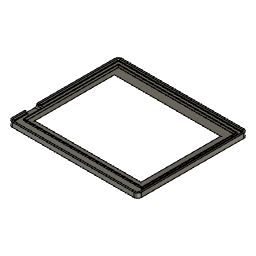
Soldered Inkplate 6Color v1.2.0. Case (Autodesk Fusion 360 archive; units mm, degrees)
design "Inkplate 6Color v1.2.0. Top"
Autodesk Fusion 360 part; units mm, degrees
sketch "Sketch1" plane through (0, 0, 0) normal (0, 0, 1) x (1, 0, 0)
  line L0 (70.2, 58.7) -> (-70.2, 58.7)
  line L1 (-70.2, 58.7) -> (-70.2, -60.7)
  line L2 (-70.2, -60.7) -> (70.2, -60.7)
  line L3 (70.2, -60.7) -> (70.2, 58.7)
  line L4 (0, 0) -> (0, -1) construction
  line L5 (58.2, 42.8) -> (-58.2, 42.8)
  line L6 (-58.2, 42.8) -> (-58.2, -44.8)
  line L7 (-58.2, -44.8) -> (58.2, -44.8)
  line L8 (58.2, -44.8) -> (58.2, 42.8)
  line L9 (58.2, 42.8) -> (-58.2, -44.8) construction
  line L10 (-58.2, 42.8) -> (58.2, -44.8) construction
  line L11 (-63.45, 47.4) -> (63.45, 47.4)
  line L12 (63.45, 47.4) -> (63.45, -52.1)
  line L13 (63.45, -52.1) -> (-63.45, -52.1)
  line L14 (-63.45, -52.1) -> (-63.45, 47.4)
  line L15 (57.6, 42.8) -> (57.6, -44.8)
  line L16 (58.2, 42.15) -> (-58.2, 42.15)
  line L17 (58.2, -44.5) -> (-58.2, -44.5)
  line L18 (-57.95, -44.8) -> (-57.95, 42.8)
  point P0 (0, -1)
  dimension "d1" = 140.4
  dimension "d55" = 1
  dimension "d56" = 116.4
  dimension "d57" = 87.6
  dimension "d58" = 15.9
  dimension "d59" = 15.9
  dimension "d60" = 119.4
  dimension "d61" = 4.6
  dimension "d62" = 5.25
  dimension "d63" = 5.25
  dimension "d64" = 99.5
  dimension "d67" = 0.6
  dimension "d68" = 0.65
  dimension "d69" = 0.25
  dimension "d70" = 0.3
  constraint horizontal L0
  constraint perpendicular L0 L1
  constraint parallel L0 L2
  constraint parallel L1 L3
  constraint coincident L4.start origin
  constraint vertical L4
  constraint horizontal L5
  constraint perpendicular L5 L6
  constraint parallel L5 L7
  constraint parallel L6 L8
  constraint coincident L9 P0
  constraint coincident L10 P0
  constraint coincident P0 L4.end
  constraint horizontal L11
  constraint vertical L12
  constraint horizontal L13
  constraint vertical L14
  constraint coincident L5 L15.start
  constraint coincident L7 L15.end
  constraint perpendicular L7 L15
  constraint coincident L8 L16.start
  constraint coincident L6 L16.end
  constraint perpendicular L6 L16
  constraint coincident L8 L17.start
  constraint coincident L6 L17.end
  constraint perpendicular L6 L17
  constraint coincident L7 L18.start
  constraint coincident L5 L18.end
  constraint perpendicular L5 L18
  measures "d1" distance of L1.end L2.end
  measures "d55" distance of L4.start P0
  measures "d56" distance of L6.end L7.end
  measures "d57" distance of L5.end L6.end
  measures "d58" distance of L0 L5
  measures "d59" distance of L2 L7
  measures "d60" distance of L0.end L1.end
  measures "d61" distance of L5 L11
  measures "d62" distance of L6 L14
  measures "d63" distance of L8 L12
  measures "d64" distance of L11.start L13.end
  measures "d67" distance of L8 L15
  measures "d68" distance of L5 L16
  measures "d69" distance of L6 L18
  measures "d70" distance of L7 L17
extrude "Extrude1" add sketch "Sketch1" along normal blind 5 contours L0 L1 L2 L3 | L5 L8 L15 L16 | L5 L15 L16 L18 | L8 L15 L16 L17 | L5 L6 L16 L18 | L7 L8 L15 L17 | L6 L16 L17 L18 | L7 L15 L17 L18 | L6 L7 L17 L18 | L11 L12 L13 L14
sketch "Sketch2" plane through (0, 0, 5) normal (0, 0, 1) x (-1, 0, 0)
  line L0 (70.2, 60.7) -> (-70.2, 60.7)
  line L1 (68.6, -57.1) -> (-68.6, -57.1)
  line L2 (-68.6, -57.1) -> (-68.6, 59.1)
  line L3 (-68.6, 59.1) -> (68.6, 59.1)
  line L4 (68.6, 59.1) -> (68.6, -57.1)
  line L5 (70.2, -58.7) -> (70.2, 60.7)
  line L6 (-70.2, -58.7) -> (70.2, -58.7)
  line L7 (-70.2, 60.7) -> (-70.2, -58.7)
  dimension "d71" = 1.6
  dimension "d72" = 1.6
  dimension "d73" = 1.6
  dimension "d74" = 1.6
  constraint horizontal L1
  constraint vertical L2
  constraint horizontal L3
  constraint vertical L4
  measures "d71" distance of L4 L5
  measures "d72" distance of L1 L6
  measures "d73" distance of L2 L7
  measures "d74" distance of L0 L3
extrude "Extrude2" cut sketch "Sketch2" against normal blind 3 contours L1 L2 L3 L4
chamfer "Chamfer1" distance 2 angle 45 4 edges at (-0.175, 42.15, 0) (57.6, -1.175, 0) (-0.175, -44.5, 0) (-57.95, -1.175, 0)
fillet "Fillet1" radius 4 4 edges at (70.2, -60.7, 2.5) (-70.2, -60.7, 2.5) (-70.2, 58.7, 2.5) (70.2, 58.7, 2.5)
sketch "Sketch3" plane through (0, 0, 2) normal (0, 0, 1) x (-1, 0, 0)
  line L0 (62.7, 42.95) -> (65.5, 42.95)
  line L1 (65.5, 42.95) -> (65.5, 29.95)
  line L2 (65.5, 29.95) -> (62.7, 29.95)
  line L3 (62.7, 29.95) -> (62.7, 42.95)
  line L4 (66.2, 60.7) -> (-66.2, 60.7)
  line L5 (65.5, 29.95) -> (68.7, 29.95)
  line L6 (68.7, 29.95) -> (68.7, 27.95)
  line L7 (68.7, 27.95) -> (65.5, 27.95)
  line L8 (65.5, 27.95) -> (65.5, 29.95)
  line L9 (62.7, 29.95) -> (65.5, 29.95)
  line L10 (65.5, 29.95) -> (65.5, 27.95)
  line L11 (65.5, 27.95) -> (62.7, 27.95)
  line L12 (62.7, 27.95) -> (62.7, 29.95)
  line L13 (62.7, 42.95) -> (65.5, 42.95)
  line L14 (65.5, 42.95) -> (65.5, 44.95)
  line L15 (65.5, 44.95) -> (62.7, 44.95)
  line L16 (62.7, 44.95) -> (62.7, 42.95)
  line L17 (57.95, -42.15) -> (-57.6, -42.15)
  line L18 (-57.6, -42.15) -> (-57.6, 44.5)
  line L19 (57.95, 44.5) -> (57.95, -42.15)
  line L20 (-57.6, 44.5) -> (57.95, 44.5)
  line L21 (68.6, 59.1) -> (-68.6, 59.1)
  line L22 (-68.6, 59.1) -> (-68.6, -57.1)
  line L23 (-68.6, -57.1) -> (68.6, -57.1)
  line L24 (68.6, -57.1) -> (68.6, 59.1)
  dimension "d15" = 13
  dimension "d16" = 17.75
  dimension "d20" = 2
  dimension "d21" = 2
  constraint horizontal L0
  constraint vertical L1
  constraint horizontal L2
  constraint vertical L3
  constraint horizontal L5
  constraint vertical L6
  constraint horizontal L7
  constraint vertical L8
  constraint horizontal L9
  constraint vertical L10
  constraint horizontal L11
  constraint vertical L12
  constraint horizontal L13
  constraint vertical L14
  constraint horizontal L15
  constraint vertical L16
  measures "d15" distance of L0.start L2.end
  measures "d16" distance of L0 L4
  measures "d20" distance of L5 L7
  measures "d21" distance of L0.start L15.end
extrude "Extrude3" add sketch "Sketch3" along normal blind 1.3 contours L0 L13 L14 L15 L16 | L0 L1 L2 L3 L9 L13 | L2 L8 L9 L10 L11 L12 | L5 L7 L8 L10 L24 | L5 L6 L7 L24
sketch "Sketch4" plane through (-70.2, 0, 0) normal (-1, 0, 0) x (0, -1, 0)
  line L0 (-54.7, 5) -> (-54.7, 0)
  line L1 (-54.7, 0) -> (56.7, 0)
  line L2 (56.7, 0) -> (56.7, 5)
  line L3 (56.7, 5) -> (-54.7, 5)
  line L4 (29.95, 5) -> (42.95, 5)
  line L5 (42.95, 5) -> (42.95, 2)
  line L6 (42.95, 2) -> (29.95, 2)
  line L7 (29.95, 2) -> (29.95, 5)
  line L8 (60.7, 0) -> (60.7, 5)
  dimension "d24" = 13
  dimension "d25" = 3
  dimension "d26" = 17.75
  constraint horizontal L4
  constraint vertical L5
  constraint horizontal L6
  constraint vertical L7
  constraint coincident L3 L4.start
  measures "d24" distance of L4.start L4.end
  measures "d25" distance of L4.start L6.end
  measures "d26" distance of L5 L8
extrude "Extrude4" cut sketch "Sketch4" against normal blind 10.5 contours L3 L4 L5 L6 L7
sketch "Sketch5" plane through (0, 0, 2) normal (0, 0, 1) x (-1, 0, 0)
  line L0 (65.5, 44.95) -> (65.5, 42.95)
  line L1 (62.7, 29.95) -> (70.2, 29.95)
  line L2 (70.2, 29.95) -> (70.2, 42.95)
  line L3 (65.5, 42.95) -> (62.7, 42.95)
  line L4 (68.6, 27.95) -> (62.7, 27.95)
  line L5 (62.7, 42.95) -> (62.7, 44.95)
  line L6 (62.7, 48.3) -> (-62.7, 48.3)
  line L7 (-62.7, 48.3) -> (-62.7, -48.3)
  line L8 (-62.7, -48.3) -> (62.7, -48.3)
  line L9 (62.7, -48.3) -> (62.7, 48.3)
  line L10 (62.7, 48.3) -> (-62.7, -48.3) construction
  line L11 (-62.7, 48.3) -> (62.7, -48.3) construction
  line L12 (64.7, 50.3) -> (-64.7, 50.3)
  line L13 (-64.7, 50.3) -> (-64.7, -50.3)
  line L14 (-64.7, -50.3) -> (64.7, -50.3)
  line L15 (64.7, -50.3) -> (64.7, 50.3)
  line L16 (64.7, 50.3) -> (-64.7, -50.3) construction
  line L17 (-64.7, 50.3) -> (64.7, -50.3) construction
  line L18 (62.7, 44.95) -> (65.5, 44.95)
  line L19 (-64.7, -51.2) -> (64.7, -51.2)
  line L20 (64.7, -51.2) -> (64.7, 51.2)
  line L21 (64.7, 51.2) -> (-64.7, 51.2)
  line L22 (-64.7, 51.2) -> (-64.7, -51.2)
  line L23 (-64.7, -51.2) -> (64.7, 51.2) construction
  line L24 (64.7, -51.2) -> (-64.7, 51.2) construction
  line L25 (-64.7, -51.2) -> (64.7, -51.2)
  line L26 (64.7, -51.2) -> (64.7, -53.2)
  line L27 (64.7, -53.2) -> (-64.7, -53.2)
  line L28 (-64.7, -53.2) -> (-64.7, -51.2)
  line L29 (-62.7, -48.3) -> (-62.7, -51.2)
  line L30 (62.7, -48.3) -> (62.7, -51.2)
  line L31 (57.95, -42.15) -> (-57.6, -42.15)
  line L32 (-57.6, -42.15) -> (-57.6, 44.5)
  line L33 (57.95, 44.5) -> (57.95, -42.15)
  line L34 (-57.6, 44.5) -> (57.95, 44.5)
  line L35 (70.2, 42.95) -> (68.6, 42.95)
  line L36 (68.6, 42.95) -> (68.6, 59.1)
  line L37 (68.6, 59.1) -> (-68.6, 59.1)
  line L38 (-68.6, 59.1) -> (-68.6, -57.1)
  line L39 (-68.6, -57.1) -> (68.6, -57.1)
  line L40 (68.6, -57.1) -> (68.6, 27.95)
  line L41 (62.7, 27.95) -> (62.7, 29.95)
  dimension "d31" = 2
  dimension "d32" = 2
  dimension "d38" = 2
  constraint horizontal L6
  constraint perpendicular L6 L7
  constraint parallel L6 L8
  constraint parallel L7 L9
  constraint coincident L10 origin
  constraint coincident L11 origin
  constraint horizontal L12
  constraint perpendicular L12 L13
  constraint parallel L12 L14
  constraint parallel L13 L15
  constraint coincident L16 origin
  constraint coincident L17 origin
  constraint horizontal L19
  constraint perpendicular L19 L20
  constraint parallel L19 L21
  constraint parallel L20 L22
  constraint coincident L23 origin
  constraint coincident L24 origin
  constraint coincident L13 L19.start
  constraint horizontal L25
  constraint vertical L26
  constraint horizontal L27
  constraint vertical L28
  constraint coincident L15 L26.end
  constraint coincident L19 L29.end
  constraint perpendicular L19 L29
  constraint coincident L25 L30.end
  constraint perpendicular L25 L30
  measures "d31" distance of L6 L12
  measures "d32" distance of L9 L15
  measures "d38" distance of L19.start L27.end
extrude "Extrude5" add sketch "Sketch5" along normal blind 1.3 contours L6 L7 L9 L12 L13 L14 L15 L18 L20 L22 L29 | L3 L5 L9 L15 L18 L20 | L1 L3 L9 L15 L20 | L4 L9 L14 L15 L20 L30 | L14 L19 L22 L25 L29 | L14 L19 L20 L25 L30 | L19 L25 L26 L27 L28
fillet "Fillet2" radius 2 3 edges at (-69.4, -42.95, 2) (-67.45, -29.95, 2) (-65.1, -42.95, 2)
chamfer "Chamfer2" distance 1.3 distance2 1.2 4 edges at (0, -48.3, 3.3) (62.7, 1.45, 3.3) (0, 51.2, 3.3) (-62.7, 1.45, 3.3) measured on face at (-63.3667, -6.5667, 3.3) measured on face at (-63.3667, -6.5667, 3.3) measured on face at (-63.3667, -6.5667, 3.3) measured on face at (-63.3667, -6.5667, 3.3)
ref_plane "WorkPlane1" through (-0.8, -1, 2.5) normal (0, 0, 1) x (1, 0, 0)
sketch "Sketch6" plane through (-0.75, 0, 2.5) normal (0, 0, 1) x (1, 0, 0)
  line L0 (-70.3196, -27.95) -> (-60.5, -27.95) construction
  line L1 (-63.95, -27.95) -> (-67.85, -27.95)
  line L2 (-67.85, -27.95) -> (-66.85, -27.95)
  line L3 (-66.85, -27.95) -> (-66.85, 55.1)
  line L4 (-66.85, 57.2) -> (-67.85, 57.2)
  line L5 (-67.85, 57.2) -> (-67.85, -27.95)
  line L6 (67.35, 56.1) -> (-65.85, 56.1)
  line L7 (-67.9314, 56.1) -> (-67.9314, 57.1)
  line L8 (68.35, 55.1) -> (68.35, -57.1)
  line L9 (-65.85, -58.1) -> (67.35, -58.1)
  line L10 (69.35, -58.1) -> (69.35, -59.1)
  line L11 (-66.85, -57.1) -> (-66.85, -43.95)
  line L12 (-66.85, -43.95) -> (-67.85, -43.95)
  line L13 (-67.85, -43.95) -> (-67.85, -59.1)
  arc A0 (-66.85, -57.1) -> (-65.85, -58.1) centre (-65.85, -57.1) ccw
  arc A1 (67.35, -58.1) -> (68.35, -57.1) centre (67.35, -57.1) ccw
  arc A2 (68.35, 55.1) -> (67.35, 56.1) centre (67.35, 55.1) ccw
  arc A3 (-65.85, 56.1) -> (-66.85, 55.1) centre (-65.85, 55.1) ccw
  line L14 (-67.85, -59.1) -> (69.35, -59.1)
  line L15 (69.35, -58.1) -> (69.35, 57.1)
  line L16 (69.35, 57.1) -> (-67.9314, 57.1)
  point P0 (-69.45, -42.95)
  point P1 (-67.85, -42.95)
  point P2 (-67.85, -59.1)
  point P3 (69.35, -59.1)
  point P4 (69.35, 57.1)
  dimension "d41" = 1
  dimension "d42" = 1
  dimension "d44" = 1
  dimension "d45" = 1
  dimension "d47" = 1
  dimension "d48" = 1
  dimension "d75" = 1
  dimension "d76" = 1
  dimension "d77" = 1
  constraint horizontal L0
  constraint coincident L0.start L1
  constraint horizontal L2
  constraint vertical L3
  constraint horizontal L4
  constraint vertical L5
  constraint coincident L1.end L2.start
  constraint horizontal L6
  constraint vertical L7
  constraint vertical L8
  constraint horizontal L9
  constraint vertical L10
  constraint vertical L11
  constraint horizontal L12
  constraint vertical L13
  constraint tangent L11 A0
  constraint tangent L9 A0
  constraint coincident L10.start L9
  constraint tangent L8 A1
  constraint tangent L9 A1
  constraint tangent L6 A2
  constraint tangent L8 A2
  constraint equal A1 A2
  constraint coincident L7.start L6
  constraint coincident L4.start L3
  constraint tangent L6 A3
  constraint tangent L3 A3
  constraint equal A1 A3
  constraint coincident P2 L13.end
  constraint coincident P3 L10.end
  constraint perpendicular L5 L16
  constraint coincident P4 L15.end
  measures "d41" distance of L1.end L2.end
  measures "d42" distance of L7.end L7.start
  measures "d44" distance of P3 L10.start
  measures "d45" distance of L11.end L12.end
  measures "d47" radius of A0
  measures "d48" radius of A1
  measures "d75" distance of L12.end P1
  measures "d76" distance of L6 L16
  measures "d77" distance of L8 L15
extrude "Extrude6" add sketch "Sketch6" along normal blind 2.5
chamfer "Chamfer3" distance 1.5 angle 45 9 edges at (-67.6, 13.575, 2.5) (-67.3071, 55.8071, 2.5) (0, 56.1, 2.5) (67.3071, 55.8071, 2.5) (67.6, -1, 2.5) (67.3071, -57.8071, 2.5) (0, -58.1, 2.5) (-67.3071, -57.8071, 2.5) (-67.6, -50.525, 2.5)
chamfer "Chamfer4" distance 1 angle 45 9 edges at (-67.6, 13.575, 5) (-67.3071, 55.8071, 5) (0, 56.1, 5) (67.3071, 55.8071, 5) (67.6, -1, 5) (67.3071, -57.8071, 5) (0, -58.1, 5) (-67.3071, -57.8071, 5) (-67.6, -50.525, 5)
equation "d57 = 85.7 mm + 1.9 mm"
